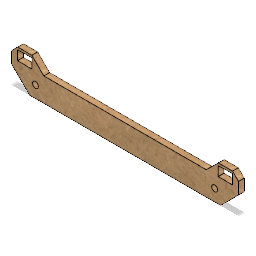
_Y endcap.e2ff004d-83c6-4757-9756-627df7789df4 (Autodesk Fusion 360 design; units mm, degrees)
Autodesk Fusion 360 part; units mm, degrees
sketch "Sketch1" plane through (0, 0, 0) normal (0, 0, 1) x (1, 0, 0)
  line L0 (100, -10) -> (-100, -10)
  line L1 (-100, -10) -> (-100, 20)
  line L2 (-100, 20) -> (100, 20)
  line L3 (100, 20) -> (100, -10)
  line L4 (0, 10) -> (-90, 10)
  line L5 (0, 10) -> (90, 10)
  line L6 (-90, 10) -> (-90, 18)
  line L7 (-90, 18) -> (-78, 18)
  line L8 (-78, 10) -> (-78, 18)
  line L9 (90, 10) -> (90, 18)
  line L10 (90, 18) -> (78, 18)
  line L11 (78, 18) -> (78, 10)
  line L12 (89.989, 20) -> (95, 15)
  line L13 (95, 15) -> (95, 5)
  line L14 (95, 5) -> (80.0328, -10)
  line L15 (-90, 20) -> (-95.0166, 14.9724)
  line L16 (-95.0166, 14.9724) -> (-95.0166, 5)
  line L17 (-95.0166, 5) -> (-79.9838, -10)
  line L18 (78, 20) -> (67.9871, 10)
  line L19 (-78, 20) -> (-68.0075, 10)
  circle A0 centre (-75, 0) radius 2.5
  circle A1 centre (75, 0) radius 2.5
  dimension "d1" = 200
  dimension "d2" = 30
  dimension "d3" = 90
  dimension "d4" = 90
  dimension "d5" = 8
  dimension "d6" = 12
  dimension "d7" = 8
  dimension "d8" = 12
  dimension "d9" = 5
  dimension "d10" = 5
  constraint horizontal L0
  constraint vertical L1
  constraint horizontal L2
  constraint vertical L3
  constraint horizontal L4
  constraint parallel L4 L5
  constraint perpendicular L4 L6
  constraint perpendicular L6 L7
  constraint coincident L4 L8.start
  constraint perpendicular L7 L8
  constraint perpendicular L5 L9
  constraint perpendicular L9 L10
  constraint coincident L5 L11.end
  constraint perpendicular L5 L11
  constraint coincident L2 L12.start
  constraint parallel L3 L13
  constraint coincident L0 L14.end
  constraint perpendicular L12 L14
  constraint coincident L2 L15.start
  constraint parallel L14 L15
  constraint perpendicular L2 L16
  constraint coincident L0 L17.end
  constraint perpendicular L15 L17
  constraint coincident L2 L18.start
  constraint coincident L5 L18.end
  constraint coincident L2 L19.start
  constraint coincident L4 L19.end
  measures "d1" distance of L0.start L0.end
  measures "d2" distance of L0.start L2.end
  measures "d3" distance of L4.start L4.end
  measures "d4" distance of L4.start L5.end
  measures "d5" distance of L4.end L6.end
  measures "d6" distance of L6.end L7.end
  measures "d7" distance of L5.end L9.end
  measures "d8" distance of L9.end L10.end
  measures "d9" diameter of A0
  measures "d10" diameter of A1
extrude "Extrude1" add sketch "Sketch1" along normal blind 5 contours L0 L2 L4 L5 L12 L13 L14 L15 L16 L17 L18 L19
sketch "Sketch2" plane through (0, 0, 5) normal (0, 0, 1) x (1, 0, 0)
  circle A0 centre (75, 0) radius 2.5
  circle A1 centre (-75, 0) radius 2.5
  line L0 (78, 10) -> (78, 18)
  line L1 (78, 18) -> (90, 18)
  line L2 (90, 18) -> (90, 10)
  line L3 (90, 10) -> (78, 10)
  line L4 (-78, 10) -> (-90, 10)
  line L5 (-90, 10) -> (-90, 18)
  line L6 (-90, 18) -> (-78, 18)
  line L7 (-78, 18) -> (-78, 10)
  line L8 (-90, 20) -> (-95.0166, 14.9724)
  line L9 (-95.0166, 14.9724) -> (-95.0166, 5)
  line L10 (-95.0166, 5) -> (-79.9838, -10)
  line L11 (-79.9838, -10) -> (80.0328, -10)
  line L12 (80.0328, -10) -> (95, 5)
  line L13 (95, 5) -> (95, 15)
  line L14 (95, 15) -> (89.989, 20)
  line L15 (89.989, 20) -> (78, 20)
  line L16 (78, 20) -> (67.9871, 10)
  line L17 (67.9871, 10) -> (-68.0075, 10)
  line L18 (-68.0075, 10) -> (-78, 20)
  line L19 (-78, 20) -> (-90, 20)
equation "d3 = ( 168 / 2 ) * 1 mm + 6 mm"
